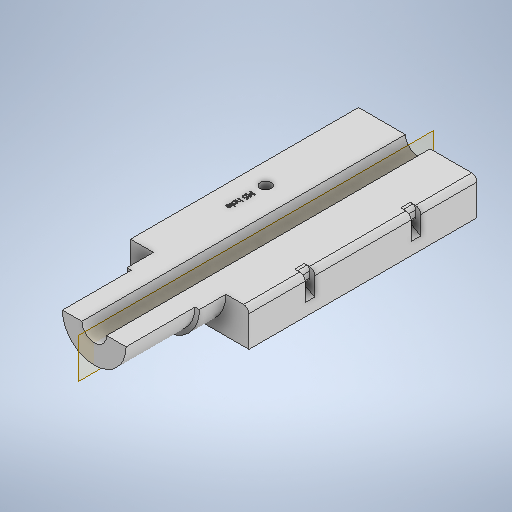
# Autodesk Inventor part: Pen_Housing_Bottom_V2
Saved by Autodesk Inventor 2025 (Build 290162000, 162)
## iProperties
Created: 2024-05-30
Part Number: Pen_Housing_Bottom_V2
Material: Generic
Document SubType Name: Modeling
Designer: mumin
Density: 1 g/cm^3
Appearance: Default
Author: mumin
Autodesk Inventor part; units mm, degrees
ref_plane "XZ Plane" through (0, 0, 0) normal (0, 1, 0) x (-1, 0, 0)
sketch "Sketch1" plane through (0, 0, 0) normal (1, 0, 0) x (0, 1, 0)
  line L0 (-20.5, -64.5) -> (0, -64.5)
  line L1 (0, -64.5) -> (0, 64.5)
  line L2 (0, 64.5) -> (-20.5, 64.5)
  line L3 (-20.5, 64.5) -> (-20.5, -64.5)
  line L4 (-20.5, -64.5) -> (0, 64.5) construction
  line L5 (0, -64.5) -> (-20.5, 64.5) construction
  line L6 (-24.6, 0) -> (4.1, 0) projected
  point P0 (0, 0)
  point P1 (-10.25, 0)
  dimension "d0" = 20.5
  dimension "d1" = 129
  constraints: 12 end point, 4 midpoint, 2 parallel, 1 horizontal, 1 perpendicular
  measures "d0" distance of L1.end L2.end
  measures "d1" distance of L2.end L0.start
extrude "Extrusion1" add sketch "Sketch1" along normal mid plane 67
sketch "Sketch2" plane through (-33.5, -20.5, 64.5) normal (0, 0, 1) x (1, 0, 0)
  line L0 (0, 20.5) -> (67, 20.5) projected
  arc A0 (13, 20.5) -> (54, 20.5) centre (33.5, 20.5) ccw
  line L1 (33.5, 20.5) -> (54, 20.5) construction
  line L2 (33.5, 20.5) -> (13, 20.5) construction
  point P0 (54, 20.5)
  dimension "d4" = 20.5
  dimension "d5" = 180
  constraints: 4 end point, 2 point on circle, 1 centre point, 1 coincident, 1 point on line
  measures "d4" radius of A0
  measures "d5" angle of L2 L1
extrude "Extrusion2" add sketch "Sketch2" along normal blind 15
sketch "Sketch3" plane through (-33.5, -20.5, 79.5) normal (0, 0, 1) x (1, 0, 0)
  line L0 (67, 20.5) -> (0, 20.5) projected
  arc A0 (15.5, 20.5) -> (51.5, 20.5) centre (33.5, 20.5) ccw
  line L1 (33.5, 20.5) -> (15.5, 20.5) construction
  line L2 (33.5, 20.5) -> (51.5, 20.5) construction
  dimension "d8" = 18
  dimension "d9" = 180
  constraints: 4 end point, 2 point on circle, 1 centre point, 1 coincident, 1 point on line
  measures "d8" radius of A0
  measures "d9" angle of L1 L2
extrude "Extrusion3" add sketch "Sketch3" along normal blind 39
sketch "Sketch4" plane through (33.5, 0, -64.5) normal (0, 0, -1) x (-1, 0, 0)
  line L0 (0, 0) -> (67, 0) projected
  arc A0 (26.5, 0) -> (40.5, 0) centre (33.5, 0) ccw
  line L1 (33.5, 0) -> (40.5, 0) construction
  line L2 (33.5, 0) -> (26.5, 0) construction
  point P0 (40.5, 0)
  dimension "d12" = 7
  dimension "d13" = 180
  constraints: 4 end point, 2 point on circle, 1 centre point, 1 coincident, 1 point on line
  measures "d12" radius of A0
  measures "d13" angle of L1 L2
extrude "Extrusion4" cut sketch "Sketch4" against normal through all
ref_plane "Work Plane1" through (0, 0, 30) normal (0, 0, 1) x (1, 0, 0)
sketch "Sketch5" plane through (0, 0, 30) normal (0, 0, 1) x (1, 0, 0)
  line L0 (33.5, -2) -> (33.5, -10.1)
  arc A0 (25.8, -8) -> (26.8834, -9.8375) centre (27.9, -8) ccw
  line L1 (25.8, -8) -> (25.8, -4.9024)
  arc A1 (27.8704, -6.2736) -> (25.8, -4.9024) centre (25.9, -7) ccw
  line L2 (28.8087, -6.9278) -> (29.3, -6.9278)
  line L3 (30.8, -5.4278) -> (30.8, -2)
  arc A2 (30.8, -2) -> (29.0387, -0.1051) centre (28.9, -2) ccw
  line L4 (29.0387, -0.1051) -> (27.6036, 0)
  line L5 (31.5, 0) -> (27.6036, 0)
  arc A3 (32.6591, -0.3701) -> (31.5, 0) centre (31.5, -2) ccw
  arc A4 (29.3, -6.9278) -> (30.8, -5.4278) centre (29.3, -5.4278) ccw
  line L6 (26.8834, -9.8375) -> (33.5, -13.4982)
  line L7 (33.5, -13.4982) -> (33.5, -10.1)
  arc A5 (27.8704, -6.2736) -> (28.8087, -6.9278) centre (28.8087, -5.9278) ccw
  line L8 (-53.4107, 0) -> (47.9851, 0) projected
  line L9 (33.5, -20.5) -> (33.5, 0) projected
  point P0 (0, 0)
  point P1 (33.4, 0)
  point P2 (33.5, 0)
  point P3 (33.5, -8)
  point P4 (31.4, -10.1)
  point P5 (27.9988, -6.9278)
  point P6 (30.8, -6.9278)
  point P7 (31.5, 0)
  dimension "d17" = 2
  dimension "d18" = 1.5
  dimension "d19" = 1
  constraints: 16 end point, 13 point on circle, 8 tangent, 7 point on line, 6 centre point, 1 collinear
  measures "d17" radius of A3
  measures "d18" radius of A4
  measures "d19" radius of A5
extrude "Extrusion5" cut sketch "Sketch5" along normal mid plane 5.4
mirror "Mirror1" about plane through (0, 0, 0) normal (0, 0, 1) of "Extrusion5"
fillet "Fillet1" radius 3 3 edges at (33.5, 0, 48.6) (33.5, 0, 0) (33.5, 0, -48.6)
sketch "Sketch6" plane through (-33.5, 0, 64.5) normal (0, 1, 0) x (1, 0, 0)
  line L0 (80.4, 64.5) -> (-13.4, 64.5) projected
  line L1 (0, 0) -> (0, 129) projected
  point P0 (33.5, 64.5)
  point P1 (12, 64.5)
  dimension "d30" = 12
  constraints: 1 point on line
  measures "d30" distance from line of L1 point (12, 64.5)
hole "Hole1" at (-21.5, 0, 0) direction (0, -1, 0) diameter 6.2 depth 10
sketch "Sketch7" plane through (-33.5, 0, 64.5) normal (0, 1, 0) x (1, 0, 0)
  line L0 (13.549, 57.6573) -> (13.549, 43.0546) construction
  line L1 (13.549, 43.0546) -> (10.1361, 43.0546) construction
  line L2 (10.1361, 43.0546) -> (10.1361, 57.6573) construction
  line L3 (10.1361, 57.6573) -> (13.549, 57.6573) construction
  line L4 (10.3652, 54.7353) -> (10.3652, 55.1404)
  line L5 (10.3652, 55.1404) -> (12.9908, 55.1404)
  line L6 (12.9908, 55.1404) -> (11.205, 55.9357)
  line L7 (11.205, 55.9357) -> (11.205, 56.1827)
  line L8 (11.205, 56.1827) -> (12.9908, 56.9707)
  line L9 (12.9908, 56.9707) -> (10.3652, 56.9707)
  line L10 (10.3652, 56.9707) -> (10.3652, 57.3486)
  line L11 (10.3652, 57.3486) -> (13.4132, 57.3486)
  line L12 (13.4132, 57.3486) -> (13.4132, 56.7953)
  line L13 (13.4132, 56.7953) -> (11.7163, 56.0345)
  line L14 (11.7163, 56.0345) -> (13.4132, 55.2984)
  line L15 (13.4132, 55.2984) -> (13.4132, 54.7353)
  line L16 (13.4132, 54.7353) -> (10.3652, 54.7353)
  spline S0 degree 2 poles (11.3532, 52.2776) (11.1185, 52.2776) (10.7209, 52.4332) (10.5875, 52.5641) knots 0 0 0 1 2 2 2
  spline S1 degree 2 poles (10.5875, 52.5641) (10.4467, 52.7) (10.301, 53.0409) (10.301, 53.2459) knots 0 0 0 1 2 2 2
  spline S2 degree 2 poles (10.301, 53.2459) (10.301, 53.4509) (10.4393, 53.7893) (10.5776, 53.9177) knots 0 0 0 1 2 2 2
  spline S3 degree 2 poles (10.5776, 53.9177) (10.7431, 54.0758) (11.2989, 54.2536) (11.7039, 54.2536) knots 0 0 0 1 2 2 2
  spline S4 degree 2 poles (11.7039, 54.2536) (12.1016, 54.2536) (12.7413, 54.0906) (12.9785, 53.9202) knots 0 0 0 1 2 2 2
  spline S5 degree 2 poles (12.9785, 53.9202) (13.2106, 53.7547) (13.47, 53.231) (13.47, 52.8877) knots 0 0 0 1 2 2 2
  spline S6 degree 2 poles (13.47, 52.8877) (13.47, 52.7864) (13.4502, 52.6086) (13.428, 52.5419) knots 0 0 0 1 2 2 2
  line L17 (13.428, 52.5419) -> (13.0353, 52.5419)
  line L18 (13.0353, 52.5419) -> (13.0353, 52.5592)
  spline S7 degree 2 poles (13.0353, 52.5592) (13.0649, 52.616) (13.1168, 52.8235) (13.1168, 52.9421) knots 0 0 0 1 2 2 2
  spline S8 degree 2 poles (13.1168, 52.9421) (13.1168, 53.3224) (12.603, 53.7893) (12.0991, 53.8337) knots 0 0 0 1 2 2 2
  spline S9 degree 2 poles (12.0991, 53.8337) (12.2004, 53.688) (12.3116, 53.3817) (12.3116, 53.1989) knots 0 0 0 1 2 2 2
  spline S10 degree 2 poles (12.3116, 53.1989) (12.3116, 53.0211) (12.2399, 52.7543) (12.1313, 52.6086) knots 0 0 0 1 2 2 2
  spline S11 degree 2 poles (12.1313, 52.6086) (12.0053, 52.4406) (11.615, 52.2776) (11.3532, 52.2776) knots 0 0 0 1 2 2 2
  spline S12 degree 2 poles (11.3359, 52.6926) (11.5236, 52.6926) (11.778, 52.7914) (11.867, 52.9001) knots 0 0 0 1 2 2 2
  spline S13 degree 2 poles (11.867, 52.9001) (11.9312, 52.9816) (11.9732, 53.1841) (11.9732, 53.2903) knots 0 0 0 1 2 2 2
  spline S14 degree 2 poles (11.9732, 53.2903) (11.9732, 53.4336) (11.8867, 53.7028) (11.8052, 53.8337) knots 0 0 0 1 2 2 2
  spline S15 degree 2 poles (11.8052, 53.8337) (11.7607, 53.8362) (11.6768, 53.8411) (11.6125, 53.8411) knots 0 0 0 1 2 2 2
  spline S16 degree 2 poles (11.6125, 53.8411) (11.2964, 53.8411) (10.9086, 53.7176) (10.8073, 53.6238) knots 0 0 0 1 2 2 2
  spline S17 degree 2 poles (10.8073, 53.6238) (10.711, 53.5373) (10.6344, 53.3496) (10.6344, 53.2434) knots 0 0 0 1 2 2 2
  spline S18 degree 2 poles (10.6344, 53.2434) (10.6344, 52.9964) (10.9852, 52.6926) (11.3359, 52.6926) knots 0 0 0 1 2 2 2
  line L19 (10.3652, 48.7554) -> (10.3652, 49.1407)
  line L20 (10.3652, 49.1407) -> (11.6694, 49.1407)
  spline S19 degree 2 poles (11.6694, 49.1407) (11.8274, 49.1407) (12.0991, 49.1703) (12.1807, 49.2148) knots 0 0 0 1 2 2 2
  spline S20 degree 2 poles (12.1807, 49.2148) (12.2671, 49.2617) (12.3511, 49.4297) (12.3511, 49.573) knots 0 0 0 1 2 2 2
  spline S21 degree 2 poles (12.3511, 49.573) (12.3511, 49.7162) (12.1979, 50.02) (12.0744, 50.1658) knots 0 0 0 1 2 2 2
  line L21 (12.0744, 50.1658) -> (10.3652, 50.1658)
  line L22 (10.3652, 50.1658) -> (10.3652, 50.5511)
  line L23 (10.3652, 50.5511) -> (13.549, 50.5511)
  line L24 (13.549, 50.5511) -> (13.549, 50.1658)
  line L25 (13.549, 50.1658) -> (12.398, 50.1658)
  spline S22 degree 2 poles (12.398, 50.1658) (12.5536, 49.9929) (12.7166, 49.6594) (12.7166, 49.4717) knots 0 0 0 1 2 2 2
  spline S23 degree 2 poles (12.7166, 49.4717) (12.7166, 49.1358) (12.272, 48.7554) (11.8497, 48.7554) knots 0 0 0 1 2 2 2
  line L26 (11.8497, 48.7554) -> (10.3652, 48.7554)
  spline S24 degree 2 poles (11.5088, 46.3348) (10.9308, 46.3348) (10.301, 46.8905) (10.301, 47.3549) knots 0 0 0 1 2 2 2
  spline S25 degree 2 poles (10.301, 47.3549) (10.301, 47.8316) (10.9506, 48.3775) (11.5088, 48.3775) knots 0 0 0 1 2 2 2
  spline S26 degree 2 poles (11.5088, 48.3775) (12.0818, 48.3775) (12.7166, 47.8143) (12.7166, 47.3549) knots 0 0 0 1 2 2 2
  spline S27 degree 2 poles (12.7166, 47.3549) (12.7166, 46.8905) (12.0843, 46.3348) (11.5088, 46.3348) knots 0 0 0 1 2 2 2
  spline S28 degree 2 poles (11.5088, 46.7324) (11.9534, 46.7324) (12.3857, 47.056) (12.3857, 47.3549) knots 0 0 0 1 2 2 2
  spline S29 degree 2 poles (12.3857, 47.3549) (12.3857, 47.6537) (11.9534, 47.9798) (11.5088, 47.9798) knots 0 0 0 1 2 2 2
  spline S30 degree 2 poles (11.5088, 47.9798) (11.0766, 47.9798) (10.632, 47.6537) (10.632, 47.3549) knots 0 0 0 1 2 2 2
  spline S31 degree 2 poles (10.632, 47.3549) (10.632, 47.0585) (11.0691, 46.7324) (11.5088, 46.7324) knots 0 0 0 1 2 2 2
  line L27 (10.3652, 45.5468) -> (10.3652, 45.9321)
  line L28 (10.3652, 45.9321) -> (13.549, 45.9321)
  line L29 (13.549, 45.9321) -> (13.549, 45.5468)
  line L30 (13.549, 45.5468) -> (10.3652, 45.5468)
  spline S32 degree 2 poles (10.3133, 43.9882) (10.3133, 44.5366) (10.9284, 45.1393) (11.4965, 45.1393) knots 0 0 0 1 2 2 2
  spline S33 degree 2 poles (11.4965, 45.1393) (12.0547, 45.1393) (12.7166, 44.5539) (12.7166, 44.0821) knots 0 0 0 1 2 2 2
  spline S34 degree 2 poles (12.7166, 44.0821) (12.7166, 43.8697) (12.5931, 43.5412) (12.4622, 43.4201) knots 0 0 0 1 2 2 2
  spline S35 degree 2 poles (12.4622, 43.4201) (12.3313, 43.2966) (11.9534, 43.1657) (11.6792, 43.1657) knots 0 0 0 1 2 2 2
  line L31 (11.6792, 43.1657) -> (11.4693, 43.1657)
  line L32 (11.4693, 43.1657) -> (11.4693, 44.749)
  spline S36 degree 2 poles (11.4693, 44.749) (11.0716, 44.749) (10.6492, 44.3489) (10.6492, 43.9932) knots 0 0 0 1 2 2 2
  spline S37 degree 2 poles (10.6492, 43.9932) (10.6492, 43.8672) (10.7061, 43.6227) (10.7505, 43.5239) knots 0 0 0 1 2 2 2
  spline S38 degree 2 poles (10.7505, 43.5239) (10.7999, 43.4201) (10.8864, 43.2769) (10.9259, 43.2299) knots 0 0 0 1 2 2 2
  line L33 (10.9259, 43.2299) -> (10.9259, 43.2077)
  line L34 (10.9259, 43.2077) -> (10.506, 43.2077)
  spline S39 degree 2 poles (10.506, 43.2077) (10.4788, 43.2744) (10.3998, 43.477) (10.3775, 43.556) knots 0 0 0 1 2 2 2
  spline S40 degree 2 poles (10.3775, 43.556) (10.3454, 43.6671) (10.3133, 43.8499) (10.3133, 43.9882) knots 0 0 0 1 2 2 2
  spline S41 degree 2 poles (11.7632, 43.5412) (11.9188, 43.5461) (12.1461, 43.6103) (12.2226, 43.6721) knots 0 0 0 1 2 2 2
  spline S42 degree 2 poles (12.2226, 43.6721) (12.3091, 43.7388) (12.4005, 43.9487) (12.4005, 44.1043) knots 0 0 0 1 2 2 2
  spline S43 degree 2 poles (12.4005, 44.1043) (12.4005, 44.2575) (12.3091, 44.4724) (12.2202, 44.5613) knots 0 0 0 1 2 2 2
  spline S44 degree 2 poles (12.2202, 44.5613) (12.1288, 44.6477) (11.9089, 44.7367) (11.7632, 44.749) knots 0 0 0 1 2 2 2
  line L35 (11.7632, 44.749) -> (11.7632, 43.5412)
  point P0 (33.5, 64.5)
  constraints: 2 other
emboss "Emboss1" sketch "Sketch7" operation cut depth 1 direction (0, -1, 0)
sketch "Sketch9" plane through (-33.5, -20.5, -64.5) normal (0, -1, 0) x (1, 0, 0)
  line L0 (51.5, 183) -> (15.5, 183) projected
  line L1 (33.5, 219.6) -> (33.5, -36.6) projected
  point P0 (33.5, 64.5)
  point P1 (33.5, 31)
  dimension "d54" = 152
  constraints: 1 point on line
  measures "d54" distance from line of L0 point (33.5, 31)
hole "Hole2" at (0, -20.5, -33.5) direction (0, 1, 0) diameter 5.2 depth 10
sketch "Sketch10" plane through (-33.5, -20.5, -64.5) normal (0, -1, 0) x (1, 0, 0)
  line L0 (33.5, 219.6) -> (33.5, -36.6) projected
  line L1 (51.5, 183) -> (15.5, 183) projected
  point P0 (33.5, 64.5)
  point P1 (33.5, 116)
  dimension "d55" = 67
  constraints: 1 point on line
  measures "d55" distance from line of L1 point (33.5, 116)
hole "Hole3" at (0, -20.5, 51.5) direction (0, 1, 0) diameter 5.2 depth 10
sketch "Sketch11" plane through (-33.5, -20.5, -64.5) normal (0, -1, 0) x (1, 0, 0)
  line L0 (33.5, 219.6) -> (33.5, -36.6) projected
  line L1 (51.5, 183) -> (15.5, 183) projected
  point P0 (33.5, 64.5)
  point P1 (33.5, 73)
  dimension "d56" = 110
  constraints: 1 point on line
  measures "d56" distance from line of L1 point (33.5, 73)
hole "Hole4" at (0, -20.5, 8.5) direction (0, 1, 0) diameter 6.55 depth 10
sketch "Sketch12" plane through (-33.5, -20.5, -64.5) normal (0, -1, 0) x (1, 0, 0)
  line L0 (24.1028, 28.9469) -> (24.1028, 34.465) construction
  line L1 (24.1028, 34.465) -> (27.2719, 34.465) construction
  line L2 (27.2719, 34.465) -> (27.2719, 28.9469) construction
  line L3 (27.2719, 28.9469) -> (24.1028, 28.9469) construction
  line L4 (24.9459, 113.1111) -> (24.9459, 118.6291) construction
  line L5 (24.9459, 118.6291) -> (28.115, 118.6291) construction
  line L6 (28.115, 118.6291) -> (28.115, 113.1111) construction
  line L7 (28.115, 113.1111) -> (24.9459, 113.1111) construction
  line L8 (23.2734, 66.1402) -> (23.2734, 71.6582) construction
  line L9 (23.2734, 71.6582) -> (26.4424, 71.6582) construction
  line L10 (26.4424, 71.6582) -> (26.4424, 66.1402) construction
  line L11 (26.4424, 66.1402) -> (23.2734, 66.1402) construction
  line L12 (26.4572, 68.089) -> (26.4572, 66.6021)
  line L13 (26.4572, 66.6021) -> (26.146, 66.6021)
  line L14 (26.146, 66.6021) -> (26.146, 67.1554)
  line L15 (26.146, 67.1554) -> (24.1033, 67.1554)
  line L16 (24.1033, 67.1554) -> (24.1033, 66.6021)
  line L17 (24.1033, 66.6021) -> (23.8242, 66.6021)
  spline S0 degree 2 poles (23.8242, 66.6021) (23.8242, 66.9158) (23.6464, 67.2122) (23.3994, 67.232) knots 0 0 0 1 2 2 2
  line L18 (23.3994, 67.232) -> (23.3994, 67.5481)
  line L19 (23.3994, 67.5481) -> (26.146, 67.5481)
  line L20 (26.146, 67.5481) -> (26.146, 68.089)
  line L21 (26.146, 68.089) -> (26.4572, 68.089)
  line L22 (23.2734, 69.9169) -> (27.1192, 68.7238)
  line L23 (27.1192, 68.7238) -> (27.1192, 68.378)
  line L24 (27.1192, 68.378) -> (23.2734, 69.5661)
  line L25 (23.2734, 69.5661) -> (23.2734, 69.9169)
  line L26 (25.4099, 72.214) -> (25.4099, 71.8509)
  line L27 (25.4099, 71.8509) -> (26.4572, 71.8509)
  line L28 (26.4572, 71.8509) -> (26.4572, 71.4581)
  line L29 (26.4572, 71.4581) -> (25.4099, 71.4581)
  line L30 (25.4099, 71.4581) -> (25.4099, 70.112)
  line L31 (25.4099, 70.112) -> (24.9802, 70.112)
  line L32 (24.9802, 70.112) -> (23.4092, 71.4754)
  line L33 (23.4092, 71.4754) -> (23.4092, 71.8509)
  line L34 (23.4092, 71.8509) -> (25.0814, 71.8509)
  line L35 (25.0814, 71.8509) -> (25.0814, 72.214)
  line L36 (25.0814, 72.214) -> (25.4099, 72.214)
  line L37 (25.0814, 71.4581) -> (23.8909, 71.4581)
  line L38 (23.8909, 71.4581) -> (25.0814, 70.4331)
  line L39 (25.0814, 70.4331) -> (25.0814, 71.4581)
  line L40 (25.3087, 73.6565) -> (25.3087, 72.503)
  line L41 (25.3087, 72.503) -> (24.9382, 72.503)
  line L42 (24.9382, 72.503) -> (24.9382, 73.6565)
  line L43 (24.9382, 73.6565) -> (25.3087, 73.6565)
  line L44 (26.4572, 75.9412) -> (26.4572, 74.0615)
  line L45 (26.4572, 74.0615) -> (26.025, 74.0615)
  spline S1 degree 2 poles (26.025, 74.0615) (25.8348, 74.2641) (25.4816, 74.6247) (25.2914, 74.7976) knots 0 0 0 1 2 2 2
  spline S2 degree 2 poles (25.2914, 74.7976) (24.9085, 75.1459) (24.4491, 75.4003) (24.2046, 75.4003) knots 0 0 0 1 2 2 2
  spline S3 degree 2 poles (24.2046, 75.4003) (24.0761, 75.4003) (23.8835, 75.3213) (23.8217, 75.2496) knots 0 0 0 1 2 2 2
  spline S4 degree 2 poles (23.8217, 75.2496) (23.76, 75.178) (23.6982, 74.9903) (23.6982, 74.8767) knots 0 0 0 1 2 2 2
  spline S5 degree 2 poles (23.6982, 74.8767) (23.6982, 74.768) (23.7526, 74.5457) (23.7946, 74.4444) knots 0 0 0 1 2 2 2
  spline S6 degree 2 poles (23.7946, 74.4444) (23.8291, 74.3579) (23.9279, 74.1974) (23.9625, 74.148) knots 0 0 0 1 2 2 2
  line L46 (23.9625, 74.148) -> (23.9625, 74.1258)
  line L47 (23.9625, 74.1258) -> (23.5278, 74.1258)
  spline S7 degree 2 poles (23.5278, 74.1258) (23.466, 74.2517) (23.345, 74.7037) (23.345, 74.9063) knots 0 0 0 1 2 2 2
  spline S8 degree 2 poles (23.345, 74.9063) (23.345, 75.3336) (23.797, 75.8153) (24.1823, 75.8153) knots 0 0 0 1 2 2 2
  spline S9 degree 2 poles (24.1823, 75.8153) (24.3627, 75.8153) (24.664, 75.7313) (24.7924, 75.6572) knots 0 0 0 1 2 2 2
  spline S10 degree 2 poles (24.7924, 75.6572) (24.9258, 75.5831) (25.1876, 75.3682) (25.3136, 75.2496) knots 0 0 0 1 2 2 2
  spline S11 degree 2 poles (25.3136, 75.2496) (25.5236, 75.057) (25.9731, 74.5852) (26.104, 74.4444) knots 0 0 0 1 2 2 2
  line L48 (26.104, 74.4444) -> (26.104, 75.9412)
  line L49 (26.104, 75.9412) -> (26.4572, 75.9412)
  spline S12 degree 2 poles (24.9332, 78.2458) (25.7533, 78.2458) (26.5215, 77.769) (26.5215, 77.2726) knots 0 0 0 1 2 2 2
  spline S13 degree 2 poles (26.5215, 77.2726) (26.5215, 76.7687) (25.7385, 76.2969) (24.9357, 76.2969) knots 0 0 0 1 2 2 2
  spline S14 degree 2 poles (24.9357, 76.2969) (24.1107, 76.2969) (23.3475, 76.7736) (23.3475, 77.2726) knots 0 0 0 1 2 2 2
  spline S15 degree 2 poles (23.3475, 77.2726) (23.3475, 77.774) (24.1379, 78.2458) (24.9332, 78.2458) knots 0 0 0 1 2 2 2
  spline S16 degree 2 poles (25.862, 77.7221) (25.7113, 77.7814) (25.2469, 77.8308) (24.9332, 77.8308) knots 0 0 0 1 2 2 2
  spline S17 degree 2 poles (24.9332, 77.8308) (24.6195, 77.8308) (24.1576, 77.7814) (24.002, 77.7196) knots 0 0 0 1 2 2 2
  spline S18 degree 2 poles (24.002, 77.7196) (23.8464, 77.6579) (23.6859, 77.443) (23.6859, 77.2726) knots 0 0 0 1 2 2 2
  spline S19 degree 2 poles (23.6859, 77.2726) (23.6859, 77.1021) (23.8464, 76.8823) (24.007, 76.8181) knots 0 0 0 1 2 2 2
  spline S20 degree 2 poles (24.007, 76.8181) (24.1626, 76.7563) (24.6368, 76.7119) (24.9357, 76.7119) knots 0 0 0 1 2 2 2
  spline S21 degree 2 poles (24.9357, 76.7119) (25.2568, 76.7119) (25.6866, 76.7514) (25.8546, 76.8156) knots 0 0 0 1 2 2 2
  spline S22 degree 2 poles (25.8546, 76.8156) (26.0126, 76.8749) (26.1831, 77.0947) (26.1831, 77.2726) knots 0 0 0 1 2 2 2
  spline S23 degree 2 poles (26.1831, 77.2726) (26.1831, 77.4405) (26.0225, 77.6604) (25.862, 77.7221) knots 0 0 0 1 2 2 2
  line L50 (27.2077, 31.869) -> (27.2077, 31.4639)
  line L51 (27.2077, 31.4639) -> (24.582, 31.4639)
  line L52 (24.582, 31.4639) -> (26.3678, 30.6685)
  line L53 (26.3678, 30.6685) -> (26.3678, 30.4215)
  line L54 (26.3678, 30.4215) -> (24.582, 29.6336)
  line L55 (24.582, 29.6336) -> (27.2077, 29.6336)
  line L56 (27.2077, 29.6336) -> (27.2077, 29.2557)
  line L57 (27.2077, 29.2557) -> (24.1597, 29.2557)
  line L58 (24.1597, 29.2557) -> (24.1597, 29.809)
  line L59 (24.1597, 29.809) -> (25.8566, 30.5697)
  line L60 (25.8566, 30.5697) -> (24.1597, 31.3058)
  line L61 (24.1597, 31.3058) -> (24.1597, 31.869)
  line L62 (24.1597, 31.869) -> (27.2077, 31.869)
  spline S24 degree 2 poles (26.2196, 34.3266) (26.4543, 34.3266) (26.852, 34.171) (26.9854, 34.0401) knots 0 0 0 1 2 2 2
  spline S25 degree 2 poles (26.9854, 34.0401) (27.1261, 33.9043) (27.2719, 33.5634) (27.2719, 33.3584) knots 0 0 0 1 2 2 2
  spline S26 degree 2 poles (27.2719, 33.3584) (27.2719, 33.1534) (27.1336, 32.815) (26.9952, 32.6866) knots 0 0 0 1 2 2 2
  spline S27 degree 2 poles (26.9952, 32.6866) (26.8297, 32.5285) (26.274, 32.3506) (25.8689, 32.3506) knots 0 0 0 1 2 2 2
  spline S28 degree 2 poles (25.8689, 32.3506) (25.4712, 32.3506) (24.8315, 32.5137) (24.5944, 32.6841) knots 0 0 0 1 2 2 2
  spline S29 degree 2 poles (24.5944, 32.6841) (24.3622, 32.8496) (24.1028, 33.3732) (24.1028, 33.7165) knots 0 0 0 1 2 2 2
  spline S30 degree 2 poles (24.1028, 33.7165) (24.1028, 33.8178) (24.1226, 33.9957) (24.1448, 34.0624) knots 0 0 0 1 2 2 2
  line L63 (24.1448, 34.0624) -> (24.5376, 34.0624)
  line L64 (24.5376, 34.0624) -> (24.5376, 34.0451)
  spline S31 degree 2 poles (24.5376, 34.0451) (24.5079, 33.9883) (24.4561, 33.7808) (24.4561, 33.6622) knots 0 0 0 1 2 2 2
  spline S32 degree 2 poles (24.4561, 33.6622) (24.4561, 33.2818) (24.9698, 32.815) (25.4737, 32.7705) knots 0 0 0 1 2 2 2
  spline S33 degree 2 poles (25.4737, 32.7705) (25.3724, 32.9163) (25.2613, 33.2225) (25.2613, 33.4053) knots 0 0 0 1 2 2 2
  spline S34 degree 2 poles (25.2613, 33.4053) (25.2613, 33.5832) (25.3329, 33.8499) (25.4416, 33.9957) knots 0 0 0 1 2 2 2
  spline S35 degree 2 poles (25.4416, 33.9957) (25.5676, 34.1636) (25.9578, 34.3266) (26.2196, 34.3266) knots 0 0 0 1 2 2 2
  spline S36 degree 2 poles (26.2369, 33.9117) (26.0492, 33.9117) (25.7948, 33.8129) (25.7059, 33.7042) knots 0 0 0 1 2 2 2
  spline S37 degree 2 poles (25.7059, 33.7042) (25.6417, 33.6227) (25.5997, 33.4201) (25.5997, 33.3139) knots 0 0 0 1 2 2 2
  spline S38 degree 2 poles (25.5997, 33.3139) (25.5997, 33.1707) (25.6861, 32.9014) (25.7676, 32.7705) knots 0 0 0 1 2 2 2
  spline S39 degree 2 poles (25.7676, 32.7705) (25.8121, 32.7681) (25.8961, 32.7631) (25.9603, 32.7631) knots 0 0 0 1 2 2 2
  spline S40 degree 2 poles (25.9603, 32.7631) (26.2765, 32.7631) (26.6642, 32.8866) (26.7655, 32.9805) knots 0 0 0 1 2 2 2
  spline S41 degree 2 poles (26.7655, 32.9805) (26.8619, 33.0669) (26.9384, 33.2547) (26.9384, 33.3609) knots 0 0 0 1 2 2 2
  spline S42 degree 2 poles (26.9384, 33.3609) (26.9384, 33.6079) (26.5877, 33.9117) (26.2369, 33.9117) knots 0 0 0 1 2 2 2
  line L65 (28.0507, 116.0331) -> (28.0507, 115.628)
  line L66 (28.0507, 115.628) -> (25.4251, 115.628)
  line L67 (25.4251, 115.628) -> (27.2109, 114.8327)
  line L68 (27.2109, 114.8327) -> (27.2109, 114.5857)
  line L69 (27.2109, 114.5857) -> (25.4251, 113.7977)
  line L70 (25.4251, 113.7977) -> (28.0507, 113.7977)
  line L71 (28.0507, 113.7977) -> (28.0507, 113.4198)
  line L72 (28.0507, 113.4198) -> (25.0027, 113.4198)
  line L73 (25.0027, 113.4198) -> (25.0027, 113.9731)
  line L74 (25.0027, 113.9731) -> (26.6996, 114.7339)
  line L75 (26.6996, 114.7339) -> (25.0027, 115.4699)
  line L76 (25.0027, 115.4699) -> (25.0027, 116.0331)
  line L77 (25.0027, 116.0331) -> (28.0507, 116.0331)
  spline S43 degree 2 poles (27.0627, 118.4908) (27.2974, 118.4908) (27.6951, 118.3352) (27.8284, 118.2042) knots 0 0 0 1 2 2 2
  spline S44 degree 2 poles (27.8284, 118.2042) (27.9692, 118.0684) (28.115, 117.7275) (28.115, 117.5225) knots 0 0 0 1 2 2 2
  spline S45 degree 2 poles (28.115, 117.5225) (28.115, 117.3175) (27.9766, 116.9791) (27.8383, 116.8507) knots 0 0 0 1 2 2 2
  spline S46 degree 2 poles (27.8383, 116.8507) (27.6728, 116.6926) (27.1171, 116.5148) (26.712, 116.5148) knots 0 0 0 1 2 2 2
  spline S47 degree 2 poles (26.712, 116.5148) (26.3143, 116.5148) (25.6746, 116.6778) (25.4375, 116.8482) knots 0 0 0 1 2 2 2
  spline S48 degree 2 poles (25.4375, 116.8482) (25.2053, 117.0137) (24.9459, 117.5373) (24.9459, 117.8807) knots 0 0 0 1 2 2 2
  spline S49 degree 2 poles (24.9459, 117.8807) (24.9459, 117.9819) (24.9657, 118.1598) (24.9879, 118.2265) knots 0 0 0 1 2 2 2
  line L78 (24.9879, 118.2265) -> (25.3807, 118.2265)
  line L79 (25.3807, 118.2265) -> (25.3807, 118.2092)
  spline S50 degree 2 poles (25.3807, 118.2092) (25.351, 118.1524) (25.2991, 117.9449) (25.2991, 117.8263) knots 0 0 0 1 2 2 2
  spline S51 degree 2 poles (25.2991, 117.8263) (25.2991, 117.4459) (25.8129, 116.9791) (26.3168, 116.9347) knots 0 0 0 1 2 2 2
  spline S52 degree 2 poles (26.3168, 116.9347) (26.2155, 117.0804) (26.1044, 117.3867) (26.1044, 117.5695) knots 0 0 0 1 2 2 2
  spline S53 degree 2 poles (26.1044, 117.5695) (26.1044, 117.7473) (26.176, 118.0141) (26.2847, 118.1598) knots 0 0 0 1 2 2 2
  spline S54 degree 2 poles (26.2847, 118.1598) (26.4107, 118.3277) (26.8009, 118.4908) (27.0627, 118.4908) knots 0 0 0 1 2 2 2
  spline S55 degree 2 poles (27.08, 118.0758) (26.8923, 118.0758) (26.6379, 117.977) (26.549, 117.8683) knots 0 0 0 1 2 2 2
  spline S56 degree 2 poles (26.549, 117.8683) (26.4848, 117.7868) (26.4428, 117.5843) (26.4428, 117.4781) knots 0 0 0 1 2 2 2
  spline S57 degree 2 poles (26.4428, 117.4781) (26.4428, 117.3348) (26.5292, 117.0656) (26.6107, 116.9347) knots 0 0 0 1 2 2 2
  spline S58 degree 2 poles (26.6107, 116.9347) (26.6552, 116.9322) (26.7392, 116.9272) (26.8034, 116.9272) knots 0 0 0 1 2 2 2
  spline S59 degree 2 poles (26.8034, 116.9272) (27.1196, 116.9272) (27.5073, 117.0507) (27.6086, 117.1446) knots 0 0 0 1 2 2 2
  spline S60 degree 2 poles (27.6086, 117.1446) (27.7049, 117.2311) (27.7815, 117.4188) (27.7815, 117.525) knots 0 0 0 1 2 2 2
  spline S61 degree 2 poles (27.7815, 117.525) (27.7815, 117.772) (27.4308, 118.0758) (27.08, 118.0758) knots 0 0 0 1 2 2 2
  point P0 (33.5, 64.5)
  constraints: 6 other
emboss "Emboss2" sketch "Sketch12" operation cut depth 1 direction (0, 1, 0)
body "Solid1"
